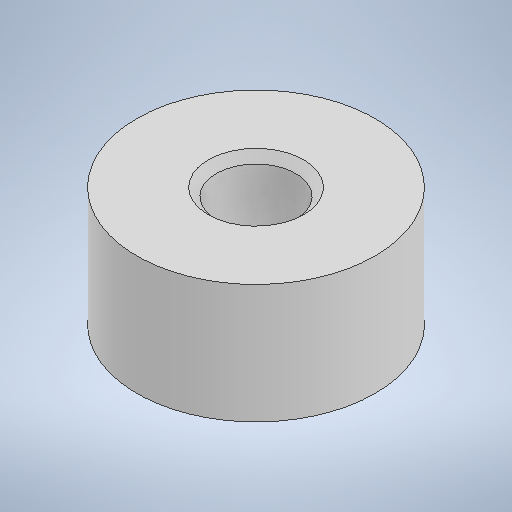
# Autodesk Inventor part: TS_Magazin_Gleitbuchse_int
Saved by Autodesk Inventor 2025.2 (Build 292293000, 293)
## iProperties
Created: 2025-06-01
Part Number: TS_Magazin_Gleitbuchse_int
Material: Generisch
Document SubType Name: Modeling
Designer: tino
Density: 1 g/cm^3
Appearance: Vorgabe
Author: tino
Autodesk Inventor part; units mm, degrees
ref_plane "YZ Plane" through (0, 0, 0) normal (1, 0, 0) x (0, 1, 0)
ref_plane "XZ Plane" through (0, 0, 0) normal (0, 1, 0) x (-1, 0, 0)
ref_plane "XY Plane" through (0, 0, 0) normal (0, 0, 1) x (1, 0, 0)
sketch "Skizze1" plane through (0, 0, 0) normal (0, 0, 1) x (1, 0, 0)
  circle A0 centre (0, 0) radius 15
  dimension "d0" = 30
  constraints: 1 centre point, 1 coincident
  measures "d0" diameter of A0
extrude "Extrusion1" add sketch "Skizze1" along normal mid plane 15
sketch "Skizze2" plane through (0, 0, 7.5) normal (0, 0, 1) x (1, 0, 0)
  point P0 (0, 0)
  point P1 (0, 0)
  constraints: 1 coincident
hole "Bohrung1" at (0, 0, 7.5) direction (0, 0, -1) diameter 10 end through all
chamfer "Fasen1" distance 1 angle 45 2 edges at (0, 5, 7.5) (0, 5, -7.5)
sketch "Skizze3" plane through (0, 0, -7.5) normal (0, 0, -1) x (-1, 0, 0)
  circle A0 centre (0, 0) radius 12.5
  circle A1 centre (0, 0) radius 7.5
  dimension "d13" = 25
  dimension "d14" = 15
  constraints: 2 centre point, 2 coincident
  measures "d13" diameter of A0
  measures "d14" diameter of A1
extrude "Extrusion2" cut sketch "Skizze3" against normal blind 10
equation "\"d0\" = Gleitbuchse_Aussendurchmesser"
equation "\"d1\" = Hoehe_Buchse"
equation "\"d3\" = Gleitbuchse_Innendurchmesser"
equation "\"d10\" = Fase"
equation "\"d13\" = Feder_aussen"
equation "\"d14\" = Feder_innen"
equation "\"d15\" = Federfuehrung_Tiefe"
equation "\"Gleitbuchse_Aussendurchmesser\" = 30"
equation "\"Gleitbuchse_Innendurchmesser\" = 10"
equation "\"Hoehe_Buchse\" = 15"
equation "\"Fase\" = 1"
equation "\"Federfuehrung_Tiefe\" = 10"
equation "\"Feder_aussen\" = 25"
equation "\"Feder_innen\" = 15"
